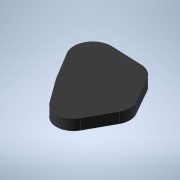
# Autodesk Inventor part: 18650_test
Saved by Autodesk Inventor 2022 (Build 260153000, 153)
## iProperties
Created: 2023-04-04
Part Number: 18650_test
Material: Типовые
Document SubType Name: Modeling
Designer: akapu
Density: 1 g/cm^3
Appearance: По умолчанию
Author: akapu
Autodesk Inventor part; units mm, degrees
ref_plane "YZ Plane" through (0, 0, 0) normal (1, 0, 0) x (0, 1, 0)
ref_plane "XZ Plane" through (0, 0, 0) normal (0, 1, 0) x (-1, 0, 0)
ref_plane "XY Plane" through (0, 0, 0) normal (0, 0, 1) x (1, 0, 0)
sketch "Эскиз1" plane through (0, 0, 0) normal (0, 1, 0) x (-1, 0, 0)
  circle A0 centre (0, 0) radius 9.25
  circle A1 centre (-8.7835, -16.5654) radius 9.5
  circle A2 centre (0.9548, -33.1704) radius 9.75
  circle A3 centre (10.7082, -15.9968) radius 10
  circle A4 centre (20.9526, -33.4643) radius 10.25
  line L0 (19.271, -10.8317) -> (29.7295, -28.1701)
  line L1 (7.4805, 5.4411) -> (18.7952, -10.1146)
  line L2 (-8.1138, 4.4418) -> (-17.1166, -12.0036)
  line L3 (-17.04, -21.2645) -> (-7.5189, -37.9932)
  line L4 (20.5459, -43.7062) -> (0.5679, -42.9128)
  line L5 (9.0979, 6.6175) -> (20.4126, -8.9381)
  line L6 (20.9836, -9.7987) -> (31.4421, -27.1371)
  circle A5 centre (20.9526, -33.4643) radius 12.25
  circle A6 centre (10.7082, -15.9968) radius 12
  circle A7 centre (0, 0) radius 11.25
  line L7 (-9.8681, 5.4022) -> (-18.8709, -11.0432)
  circle A8 centre (-8.7835, -16.5654) radius 11.5
  line L8 (-18.7781, -22.2538) -> (-9.2571, -38.9825)
  circle A9 centre (0.9548, -33.1704) radius 11.75
  line L9 (20.4665, -45.7046) -> (0.4885, -44.9112)
  point P0 (0.7124, -16.2884)
  point P1 (-3.9776, -24.7601)
  point P2 (5.7698, -24.6923)
  point P3 (10.7037, -33.3137)
  point P4 (15.7672, -24.6227)
  point P5 (5.1455, -7.6868)
  point P6 (-4.3332, -8.1723)
  point P7 (0.4885, -44.9112)
  dimension "d0" = 18.5
  dimension "d1" = 19
  dimension "d2" = 19.5
  dimension "d3" = 20
  dimension "d4" = 20.5
  dimension "d5" = 2
  dimension "d6" = 2
  dimension "d7" = 2
  dimension "d8" = 2
  dimension "d9" = 2
  dimension "d10" = 2
  dimension "d11" = 2
  dimension "d12" = 2
  dimension "d13" = 2
  dimension "d14" = 2
  constraints: 20 end point, 17 tangent, 10 centre point, 10 point on circle, 5 parallel, 1 coincident
  measures "d0" diameter of A0
  measures "d1" diameter of A1
  measures "d2" diameter of A2
  measures "d3" diameter of A3
  measures "d4" diameter of A4
  measures "d5" distance between parallel lines of L1 L5
  measures "d6" distance between parallel lines of L0 L6
  measures "d7" radial gap between concentric circles of A4 A5
  measures "d8" radial gap between concentric circles of A3 A6
  measures "d9" radial gap between concentric circles of A0 A7
  measures "d10" distance between parallel lines of L2 L7
  measures "d11" radial gap between concentric circles of A1 A8
  measures "d12" distance between parallel lines of L3 L8
  measures "d13" radial gap between concentric circles of A2 A9
  measures "d14" distance between parallel lines of L4 L9
extrude "Выдавливание1" add sketch "Эскиз1" along normal blind 5 contours A0 L1 A7 A6 | A0 L2 A7 L1 | A6 A7 A3 A0 | A0 A8 A7 L2 | A7 L5 A6 L1 | L1 A6 A7 | A3 A7 A8 A6 A0 | A6 L1 A3 A7 | A6 A8 A0 | A0 A1 A7 A8 | A7 A8 L2 | L2 A8 L7 A7 | A6 L0 A3 L1 | A3 A8 A7 | A8 A6 A7 A1 A0 | A8 A7 A6 | A7 A1 L2 A8 | L2 A1 L3 A8 | A3 A1 A6 A7 A8 | A6 A1 A7 | L0 A6 A5 A3 | L6 A5 L0 A6 | A3 A8 A9 A6 A1 | A1 A9 A8 L3 | A8 L3 A9 L8 | L0 A5 A6 | A5 L4 A4 L0 | A3 A9 A8 | A6 A9 A1 | A1 A2 A8 A9 | A8 A9 L3 | A9 L3 A2 L4 | A5 A6 A4 A3 | L0 A4 A6 A5 | A3 A2 A6 A8 A9 | A8 A6 A9 | A9 A6 A8 A2 A1 | A8 A2 L3 A9 | A9 L4 A5 L9 | A4 A6 A9 A5 A3 | A5 A9 A3 | A3 A9 A5 A6 A2 | A6 A2 A8 | A9 A5 L4 | L4 A2 A5 A9 | A4 A9 A6 | A9 A6 A5 | A5 A9 A4 L4 | A6 A5 A2 | A2 A5 A6 A9 A4 | A5 A2 A4 A9 picked at (0.4928, -9.3459) picked at (11.9874, -28.1937)
sketch "Эскиз2" plane through (0, 5, 0) normal (0, 1, 0) x (1, 0, 0)
  arc A0 (-20.9836, 9.7987) -> (-20.4126, 8.9381) centre (-10.7082, 15.9968) ccw projected
  line L0 (-20.4126, 8.9381) -> (-9.0979, -6.6175) projected
  arc A1 (-9.0979, -6.6175) -> (9.8681, -5.4022) centre (0, 0) ccw projected
  line L1 (9.8681, -5.4022) -> (18.8709, 11.0432) projected
  arc A2 (18.8709, 11.0432) -> (18.7781, 22.2538) centre (8.7835, 16.5654) ccw projected
  line L2 (18.7781, 22.2538) -> (9.2571, 38.9825) projected
  arc A3 (9.2571, 38.9825) -> (-0.4885, 44.9112) centre (-0.9548, 33.1704) ccw projected
  line L3 (-0.4885, 44.9112) -> (-20.4665, 45.7046) projected
  arc A4 (-20.4665, 45.7046) -> (-31.4421, 27.1371) centre (-20.9526, 33.4643) ccw projected
  line L4 (-31.4421, 27.1371) -> (-20.9836, 9.7987) projected
  arc A5 (-10.7037, 33.3137) -> (-15.7672, 24.6227) centre (-20.9526, 33.4643) ccw projected
  arc A6 (3.9776, 24.7601) -> (-10.7037, 33.3137) centre (-0.9548, 33.1704) ccw projected
  arc A7 (4.3332, 8.1723) -> (3.9776, 24.7601) centre (8.7835, 16.5654) ccw projected
  arc A8 (-5.1455, 7.6868) -> (4.3332, 8.1723) centre (0, 0) ccw projected
  arc A9 (-15.7672, 24.6227) -> (-5.1455, 7.6868) centre (-10.7082, 15.9968) ccw projected
  arc A10 (4.3332, 8.1723) -> (-5.1455, 7.6868) centre (0, 0) ccw projected
  arc A11 (-0.7124, 16.2884) -> (4.3332, 8.1723) centre (8.7835, 16.5654) ccw projected
  arc A12 (-5.1455, 7.6868) -> (-0.7124, 16.2884) centre (-10.7082, 15.9968) ccw projected
  arc A13 (3.9776, 24.7601) -> (-0.7124, 16.2884) centre (8.7835, 16.5654) ccw projected
  arc A14 (-5.7698, 24.6923) -> (3.9776, 24.7601) centre (-0.9548, 33.1704) ccw projected
  arc A15 (-0.7124, 16.2884) -> (-5.7698, 24.6923) centre (-10.7082, 15.9968) ccw projected
  arc A16 (-10.7037, 33.3137) -> (-5.7698, 24.6923) centre (-0.9548, 33.1704) ccw projected
  arc A17 (-15.7672, 24.6227) -> (-10.7037, 33.3137) centre (-20.9526, 33.4643) ccw projected
  arc A18 (-5.7698, 24.6923) -> (-15.7672, 24.6227) centre (-10.7082, 15.9968) ccw projected
extrude "Выдавливание2" add sketch "Эскиз2" along normal blind 2 contours L4 A4 L3 A3 L2 A2 L1 A1 L0 A0 | A17 A5 | A6 A14 A16 | A16 A18 A17 | A18 A15 A12 A9 | A7 A11 A13 | A13 A15 A14 | A10 A8 | A12 A11 A10
sketch "Эскиз3" plane through (0, 5, 0) normal (0, -1, 0) x (1, 0, 0)
  arc A0 (-5.1455, -7.6868) -> (4.3332, -8.1723) centre (0, 0) ccw projected
  arc A1 (4.3332, -8.1723) -> (-5.1455, -7.6868) centre (0, 0) ccw projected
  arc A2 (3.9776, -24.7601) -> (4.3332, -8.1723) centre (8.7835, -16.5654) ccw projected
  arc A3 (4.3332, -8.1723) -> (-0.7124, -16.2884) centre (8.7835, -16.5654) ccw projected
  arc A4 (-0.7124, -16.2884) -> (3.9776, -24.7601) centre (8.7835, -16.5654) ccw projected
  arc A5 (-5.7698, -24.6923) -> (-0.7124, -16.2884) centre (-10.7082, -15.9968) ccw projected
  arc A6 (-0.7124, -16.2884) -> (-5.1455, -7.6868) centre (-10.7082, -15.9968) ccw projected
  arc A7 (-5.1455, -7.6868) -> (-15.7672, -24.6227) centre (-10.7082, -15.9968) ccw projected
  arc A8 (-15.7672, -24.6227) -> (-5.7698, -24.6923) centre (-10.7082, -15.9968) ccw projected
  arc A9 (-5.7698, -24.6923) -> (-10.7037, -33.3137) centre (-0.9548, -33.1704) ccw projected
  arc A10 (-10.7037, -33.3137) -> (3.9776, -24.7601) centre (-0.9548, -33.1704) ccw projected
  arc A11 (3.9776, -24.7601) -> (-5.7698, -24.6923) centre (-0.9548, -33.1704) ccw projected
  arc A12 (-15.7672, -24.6227) -> (-10.7037, -33.3137) centre (-20.9526, -33.4643) ccw projected
  arc A13 (-10.7037, -33.3137) -> (-15.7672, -24.6227) centre (-20.9526, -33.4643) ccw projected
  line L0 (-5.2971, 2.241) -> (2.1639, 2.241) construction
  line L1 (2.1639, 2.241) -> (2.1639, -1.4354) construction
  line L2 (2.1639, -1.4354) -> (-5.2971, -1.4354) construction
  line L3 (-5.2971, -1.4354) -> (-5.2971, 2.241) construction
  line L4 (6.0817, -14.3017) -> (10.8583, -14.3017) construction
  line L5 (10.8583, -14.3017) -> (10.8583, -18.5083) construction
  line L6 (10.8583, -18.5083) -> (6.0817, -18.5083) construction
  line L7 (6.0817, -18.5083) -> (6.0817, -14.3017) construction
  line L8 (-6.2539, -35.262) -> (-6.2539, -31.0554) construction
  line L9 (-6.2539, -31.0554) -> (-1.4773, -31.0554) construction
  line L10 (-1.4773, -31.0554) -> (-1.4773, -35.262) construction
  line L11 (-1.4773, -35.262) -> (-6.2539, -35.262) construction
  line L12 (-13.4168, -17.9297) -> (-13.4168, -13.7231) construction
  line L13 (-13.4168, -13.7231) -> (-8.6402, -13.7231) construction
  line L14 (-8.6402, -13.7231) -> (-8.6402, -17.9297) construction
  line L15 (-8.6402, -17.9297) -> (-13.4168, -17.9297) construction
  line L16 (-26.2508, -35.3972) -> (-26.2508, -31.1906) construction
  line L17 (-26.2508, -31.1906) -> (-21.4742, -31.1906) construction
  line L18 (-21.4742, -31.1906) -> (-21.4742, -35.3972) construction
  line L19 (-21.4742, -35.3972) -> (-26.2508, -35.3972) construction
  spline S0 degree 2 poles (-2.4464, -1.59) (-2.4464, -1.6501) (-2.4652, -1.7289) (-2.4952, -1.7778) (-2.5365, -1.8003) (-2.5553, -1.8003) knots 0 0 0 1 2 3 4 4 4
  line L20 (-2.5553, -1.8003) -> (-4.6361, -1.8003)
  spline S1 degree 2 poles (-4.6361, -1.8003) (-4.6586, -1.8003) (-4.6962, -1.7778) (-4.73, -1.7289) (-4.7487, -1.6501) (-4.7487, -1.59) knots 0 0 0 1 2 3 4 4 4
  spline S2 degree 2 poles (-4.7487, -1.59) (-4.7487, -1.5374) (-4.73, -1.4548) (-4.7037, -1.4022) (-4.6624, -1.3759) (-4.6361, -1.3759) knots 0 0 0 1 2 3 4 4 4
  line L21 (-4.6361, -1.3759) -> (-3.806, -1.3759)
  line L22 (-3.806, -1.3759) -> (-3.806, 1.6551)
  line L23 (-3.806, 1.6551) -> (-4.576, 1.1969)
  spline S3 degree 2 poles (-4.576, 1.1969) (-4.6361, 1.1668) (-4.7037, 1.1556) (-4.7487, 1.1931) (-4.7638, 1.287) (-4.7638, 1.3584) knots 0 0 0 1 2 3 4 4 4
  spline S4 degree 2 poles (-4.7638, 1.3584) (-4.7638, 1.4072) (-4.7562, 1.4823) (-4.7375, 1.5311) (-4.7037, 1.5687) (-4.6736, 1.5875) knots 0 0 0 1 2 3 4 4 4
  line L24 (-4.6736, 1.5875) -> (-3.7572, 2.1734)
  spline S5 degree 2 poles (-3.7572, 2.1734) (-3.7459, 2.1847) (-3.7084, 2.1959) (-3.652, 2.2072) (-3.5769, 2.211) (-3.5243, 2.211) knots 0 0 0 1 2 3 4 4 4
  spline S6 degree 2 poles (-3.5243, 2.211) (-3.4492, 2.211) (-3.3516, 2.1997) (-3.2952, 2.1772) (-3.2764, 2.1434) (-3.2764, 2.1246) knots 0 0 0 1 2 3 4 4 4
  line L25 (-3.2764, 2.1246) -> (-3.2764, -1.3759)
  line L26 (-3.2764, -1.3759) -> (-2.5553, -1.3759)
  spline S7 degree 2 poles (-2.5553, -1.3759) (-2.5328, -1.3759) (-2.4877, -1.4022) (-2.4614, -1.4548) (-2.4464, -1.5374) (-2.4464, -1.59) knots 0 0 0 1 2 3 4 4 4
  spline S8 degree 2 poles (0.8287, -0.7787) (0.8287, -1.0379) (0.6447, -1.4397) (0.2954, -1.7177) (-0.2154, -1.8604) (-0.5422, -1.8604) knots 0 0 0 1 2 3 4 4 4
  spline S9 degree 2 poles (-0.5422, -1.8604) (-0.8501, -1.8604) (-1.3347, -1.7327) (-1.6764, -1.4773) (-1.853, -1.1092) (-1.853, -0.8726) knots 0 0 0 1 2 3 4 4 4
  spline S10 degree 2 poles (-1.853, -0.8726) (-1.853, -0.6848) (-1.729, -0.3693) (-1.4999, -0.1064) (-1.1619, 0.1265) (-0.9478, 0.2316) knots 0 0 0 1 2 3 4 4 4
  spline S11 degree 2 poles (-0.9478, 0.2316) (-1.1318, 0.3255) (-1.4173, 0.5396) (-1.6126, 0.7875) (-1.714, 1.0692) (-1.714, 1.2382) knots 0 0 0 1 2 3 4 4 4
  spline S12 degree 2 poles (-1.714, 1.2382) (-1.714, 1.4448) (-1.5638, 1.8128) (-1.2595, 2.0833) (-0.7901, 2.241) (-0.4746, 2.241) knots 0 0 0 1 2 3 4 4 4
  spline S13 degree 2 poles (-0.4746, 2.241) (-0.1741, 2.241) (0.2653, 2.0945) (0.5508, 1.8466) (0.686, 1.5086) (0.686, 1.3133) knots 0 0 0 1 2 3 4 4 4
  spline S14 degree 2 poles (0.686, 1.3133) (0.686, 1.1556) (0.5846, 0.8664) (0.3893, 0.611) (0.1038, 0.3856) (-0.0839, 0.2842) knots 0 0 0 1 2 3 4 4 4
  spline S15 degree 2 poles (-0.0839, 0.2842) (0.1376, 0.179) (0.4794, -0.0501) (0.7085, -0.313) (0.8287, -0.6059) (0.8287, -0.7787) knots 0 0 0 1 2 3 4 4 4
  spline S16 degree 2 poles (0.2916, -0.835) (0.2916, -0.6923) (0.1865, -0.4632) (-0.0239, -0.2604) (-0.3393, -0.0726) (-0.5497, 0.0288) knots 0 0 0 1 2 3 4 4 4
  spline S17 degree 2 poles (-0.5497, 0.0288) (-0.7412, -0.0689) (-1.0342, -0.2604) (-1.222, -0.4632) (-1.3159, -0.6886) (-1.3159, -0.8238) knots 0 0 0 1 2 3 4 4 4
  spline S18 degree 2 poles (-1.3159, -0.8238) (-1.3159, -1.1205) (-0.9065, -1.4473) (-0.5046, -1.4473) knots 0 0 0 1 2 2 2
  spline S19 degree 2 poles (-0.5046, -1.4473) (-0.1102, -1.4473) (0.2916, -1.1167) (0.2916, -0.835) knots 0 0 0 1 2 2 2
  spline S20 degree 2 poles (0.1639, 1.2645) (0.1639, 1.3922) (0.0738, 1.6025) (-0.099, 1.7527) (-0.3506, 1.8279) (-0.5159, 1.8279) knots 0 0 0 1 2 3 4 4 4
  spline S21 degree 2 poles (-0.5159, 1.8279) (-0.8464, 1.8279) (-1.1882, 1.5274) (-1.1882, 1.2645) knots 0 0 0 1 2 2 2
  spline S22 degree 2 poles (-1.1882, 1.2645) (-1.1882, 1.1443) (-1.1055, 0.9377) (-0.929, 0.7537) (-0.6624, 0.5772) (-0.4783, 0.4833) knots 0 0 0 1 2 3 4 4 4
  spline S23 degree 2 poles (-0.4783, 0.4833) (-0.1666, 0.6448) (0.1639, 1.0316) (0.1639, 1.2645) knots 0 0 0 1 2 2 2
  spline S24 degree 2 poles (2.2146, -1.4623) (2.2146, -1.6801) (2.0719, -1.8266) (1.8804, -1.8266) knots 0 0 0 1 2 2 2
  spline S25 degree 2 poles (1.8804, -1.8266) (1.6963, -1.8266) (1.5536, -1.6839) (1.5536, -1.4735) knots 0 0 0 1 2 2 2
  spline S26 degree 2 poles (1.5536, -1.4735) (1.5536, -1.2557) (1.7001, -1.1092) (1.8879, -1.1092) knots 0 0 0 1 2 2 2
  spline S27 degree 2 poles (1.8879, -1.1092) (2.0719, -1.1092) (2.2146, -1.2519) (2.2146, -1.4623) knots 0 0 0 1 2 2 2
  spline S28 degree 2 poles (5.5048, -0.5233) (5.5048, -0.8426) (5.2907, -1.3421) (4.8963, -1.6801) (4.3517, -1.8604) (4.0212, -1.8604) knots 0 0 0 1 2 3 4 4 4
  spline S29 degree 2 poles (4.0212, -1.8604) (3.8334, -1.8604) (3.5029, -1.8078) (3.2438, -1.7327) (3.0785, -1.6576) (3.0334, -1.6125) (3.0146, -1.5787) (2.9996, -1.5261) (2.9921, -1.4435) (2.9921, -1.3909) knots 0 0 0 1 2 3 4 5 6 7 8 8 8
  spline S30 degree 2 poles (2.9921, -1.3909) (2.9921, -1.3383) (2.9996, -1.2519) (3.0259, -1.2031) (3.0597, -1.1768) (3.0822, -1.1768) knots 0 0 0 1 2 3 4 4 4
  spline S31 degree 2 poles (3.0822, -1.1768) (3.1123, -1.1768) (3.24, -1.2557) (3.4578, -1.3458) (3.7808, -1.4247) (4.0024, -1.4247) knots 0 0 0 1 2 3 4 4 4
  spline S32 degree 2 poles (4.0024, -1.4247) (4.209, -1.4247) (4.5545, -1.3271) (4.8024, -1.1167) (4.9452, -0.8012) (4.9452, -0.5721) knots 0 0 0 1 2 3 4 4 4
  spline S33 degree 2 poles (4.9452, -0.5721) (4.9452, -0.3806) (4.825, -0.0876) (4.5771, 0.1077) (4.194, 0.2016) (3.9311, 0.2016) knots 0 0 0 1 2 3 4 4 4
  spline S34 degree 2 poles (3.9311, 0.2016) (3.7433, 0.2016) (3.4729, 0.164) (3.3564, 0.164) knots 0 0 0 1 2 2 2
  spline S35 degree 2 poles (3.3564, 0.164) (3.27, 0.164) (3.1949, 0.2429) (3.1949, 0.3593) knots 0 0 0 1 2 2 2
  line L27 (3.1949, 0.3593) -> (3.1949, 1.9819)
  spline S36 degree 2 poles (3.1949, 1.9819) (3.1949, 2.0833) (3.2888, 2.1809) (3.379, 2.1809) knots 0 0 0 1 2 2 2
  line L28 (3.379, 2.1809) -> (5.1405, 2.1809)
  spline S37 degree 2 poles (5.1405, 2.1809) (5.163, 2.1809) (5.2118, 2.1546) (5.2419, 2.0983) (5.2569, 2.0119) (5.2569, 1.9518) knots 0 0 0 1 2 3 4 4 4
  spline S38 degree 2 poles (5.2569, 1.9518) (5.2569, 1.8429) (5.1968, 1.7189) (5.1442, 1.7189) knots 0 0 0 1 2 2 2
  line L29 (5.1442, 1.7189) -> (3.7245, 1.7189)
  line L30 (3.7245, 1.7189) -> (3.7245, 0.5997)
  spline S39 degree 2 poles (3.7245, 0.5997) (3.8297, 0.6147) (4.0438, 0.6222) (4.1865, 0.6222) knots 0 0 0 1 2 2 2
  spline S40 degree 2 poles (4.1865, 0.6222) (4.517, 0.6222) (5.009, 0.4607) (5.3358, 0.1603) (5.5048, -0.2642) (5.5048, -0.5233) knots 0 0 0 1 2 3 4 4 4
  spline S41 degree 2 poles (8.9324, -18.1327) (8.9324, -18.1928) (8.9136, -18.2716) (8.8836, -18.3205) (8.8423, -18.343) (8.8235, -18.343) knots 0 0 0 1 2 3 4 4 4
  line L31 (8.8235, -18.343) -> (6.7427, -18.343)
  spline S42 degree 2 poles (6.7427, -18.343) (6.7202, -18.343) (6.6826, -18.3205) (6.6488, -18.2716) (6.6301, -18.1928) (6.6301, -18.1327) knots 0 0 0 1 2 3 4 4 4
  spline S43 degree 2 poles (6.6301, -18.1327) (6.6301, -18.0801) (6.6488, -17.9975) (6.6751, -17.9449) (6.7165, -17.9186) (6.7427, -17.9186) knots 0 0 0 1 2 3 4 4 4
  line L32 (6.7427, -17.9186) -> (7.5728, -17.9186)
  line L33 (7.5728, -17.9186) -> (7.5728, -14.8876)
  line L34 (7.5728, -14.8876) -> (6.8028, -15.3458)
  spline S44 degree 2 poles (6.8028, -15.3458) (6.7427, -15.3759) (6.6751, -15.3871) (6.6301, -15.3496) (6.615, -15.2557) (6.615, -15.1843) knots 0 0 0 1 2 3 4 4 4
  spline S45 degree 2 poles (6.615, -15.1843) (6.615, -15.1355) (6.6226, -15.0604) (6.6413, -15.0115) (6.6751, -14.974) (6.7052, -14.9552) knots 0 0 0 1 2 3 4 4 4
  line L35 (6.7052, -14.9552) -> (7.6216, -14.3693)
  spline S46 degree 2 poles (7.6216, -14.3693) (7.6329, -14.358) (7.6704, -14.3468) (7.7268, -14.3355) (7.8019, -14.3317) (7.8545, -14.3317) knots 0 0 0 1 2 3 4 4 4
  spline S47 degree 2 poles (7.8545, -14.3317) (7.9296, -14.3317) (8.0272, -14.343) (8.0836, -14.3655) (8.1024, -14.3993) (8.1024, -14.4181) knots 0 0 0 1 2 3 4 4 4
  line L36 (8.1024, -14.4181) -> (8.1024, -17.9186)
  line L37 (8.1024, -17.9186) -> (8.8235, -17.9186)
  spline S48 degree 2 poles (8.8235, -17.9186) (8.846, -17.9186) (8.8911, -17.9449) (8.9174, -17.9975) (8.9324, -18.0801) (8.9324, -18.1327) knots 0 0 0 1 2 3 4 4 4
  spline S49 degree 2 poles (12.1474, -16.1946) (12.1474, -16.4538) (12.0873, -16.9834) (11.9371, -17.4716) (11.6892, -17.8998) (11.3099, -18.2228) (10.7916, -18.4031) (10.446, -18.4031) knots 0 0 0 1 2 3 4 5 6 6 6
  spline S50 degree 2 poles (10.446, -18.4031) (10.3146, -18.4031) (10.0629, -18.3693) (9.8639, -18.3205) (9.7287, -18.2641) (9.6648, -18.2078) (9.6385, -18.1139) (9.6385, -18.035) knots 0 0 0 1 2 3 4 5 6 6 6
  spline S51 degree 2 poles (9.6385, -18.035) (9.6385, -17.9674) (9.646, -17.8848) (9.6648, -17.8435) (9.6986, -17.8284) (9.7249, -17.8284) knots 0 0 0 1 2 3 4 4 4
  spline S52 degree 2 poles (9.7249, -17.8284) (9.7587, -17.8284) (9.8826, -17.8735) (10.0704, -17.9299) (10.3221, -17.9749) (10.4798, -17.9749) knots 0 0 0 1 2 3 4 4 4
  spline S53 degree 2 poles (10.4798, -17.9749) (10.7803, -17.9749) (11.2085, -17.7458) (11.4789, -17.3552) (11.6141, -16.8482) (11.6179, -16.5627) knots 0 0 0 1 2 3 4 4 4
  spline S54 degree 2 poles (11.6179, -16.5627) (11.4564, -16.6604) (11.0019, -16.8069) (10.7052, -16.8069) knots 0 0 0 1 2 2 2
  spline S55 degree 2 poles (10.7052, -16.8069) (10.3709, -16.8069) (9.9202, -16.6266) (9.646, -16.3111) (9.5258, -15.8792) (9.5258, -15.6238) knots 0 0 0 1 2 3 4 4 4
  spline S56 degree 2 poles (9.5258, -15.6238) (9.5258, -15.3571) (9.6798, -14.8801) (10.0066, -14.5158) (10.5099, -14.3017) (10.8629, -14.3017) knots 0 0 0 1 2 3 4 4 4
  spline S57 degree 2 poles (10.8629, -14.3017) (11.1108, -14.3017) (11.4939, -14.4294) (11.7794, -14.666) (11.9747, -15.0003) (12.0949, -15.4247) (12.1474, -15.9205) (12.1474, -16.1946) knots 0 0 0 1 2 3 4 5 6 6 6
  spline S58 degree 2 poles (11.6103, -16.1383) (11.6103, -15.7439) (11.5052, -15.2031) (11.3024, -14.8688) (11.0057, -14.7223) (10.8141, -14.7223) knots 0 0 0 1 2 3 4 4 4
  spline S59 degree 2 poles (10.8141, -14.7223) (10.615, -14.7223) (10.3296, -14.8688) (10.1493, -15.1092) (10.0629, -15.4172) (10.0629, -15.5824) knots 0 0 0 1 2 3 4 4 4
  spline S60 degree 2 poles (10.0629, -15.5824) (10.0629, -15.7627) (10.138, -16.0669) (10.3108, -16.2773) (10.5888, -16.39) (10.7916, -16.39) knots 0 0 0 1 2 3 4 4 4
  spline S61 degree 2 poles (10.7916, -16.39) (11.0244, -16.39) (11.4526, -16.251) (11.6103, -16.1383) knots 0 0 0 1 2 2 2
  spline S62 degree 2 poles (-10.5736, -17.5353) (-10.5736, -17.5916) (-10.5887, -17.678) (-10.615, -17.7381) (-10.6638, -17.7644) (-10.6901, -17.7644) knots 0 0 0 1 2 3 4 4 4
  line L38 (-10.6901, -17.7644) -> (-12.891, -17.7644)
  spline S63 degree 2 poles (-12.891, -17.7644) (-12.9361, -17.7644) (-12.9999, -17.7419) (-13.045, -17.693) (-13.0675, -17.5991) (-13.0675, -17.5315) knots 0 0 0 1 2 3 4 4 4
  spline S64 degree 2 poles (-13.0675, -17.5315) (-13.0675, -17.4714) (-13.0563, -17.3775) (-13.0262, -17.3062) (-12.9774, -17.2386) (-12.9398, -17.1973) knots 0 0 0 1 2 3 4 4 4
  line L39 (-12.9398, -17.1973) -> (-12.1436, -16.3785)
  spline S65 degree 2 poles (-12.1436, -16.3785) (-11.8657, -16.0968) (-11.5314, -15.6461) (-11.3511, -15.278) (-11.2948, -14.9775) (-11.2948, -14.8423) knots 0 0 0 1 2 3 4 4 4
  spline S66 degree 2 poles (-11.2948, -14.8423) (-11.2948, -14.7109) (-11.3849, -14.4743) (-11.5539, -14.2977) (-11.8056, -14.1926) (-11.9708, -14.1926) knots 0 0 0 1 2 3 4 4 4
  spline S67 degree 2 poles (-11.9708, -14.1926) (-12.1661, -14.1926) (-12.4741, -14.2977) (-12.707, -14.4179) (-12.861, -14.5231) (-12.8985, -14.5231) knots 0 0 0 1 2 3 4 4 4
  spline S68 degree 2 poles (-12.8985, -14.5231) (-12.9211, -14.5231) (-12.9586, -14.4968) (-12.9812, -14.4442) (-12.9924, -14.3503) (-12.9924, -14.2865) knots 0 0 0 1 2 3 4 4 4
  spline S69 degree 2 poles (-12.9924, -14.2865) (-12.9924, -14.2414) (-12.9849, -14.1738) (-12.9699, -14.1212) (-12.9473, -14.0799) (-12.8722, -14.016) (-12.6919, -13.9034) (-12.4178, -13.7982) (-12.0873, -13.7231) (-11.907, -13.7231) knots 0 0 0 1 2 3 4 5 6 7 8 8 8
  spline S70 degree 2 poles (-11.907, -13.7231) (-11.6178, -13.7231) (-11.1821, -13.8846) (-10.8966, -14.17) (-10.7539, -14.5456) (-10.7539, -14.7559) knots 0 0 0 1 2 3 4 4 4
  spline S71 degree 2 poles (-10.7539, -14.7559) (-10.7539, -14.9475) (-10.8215, -15.3268) (-11.0394, -15.7663) (-11.4525, -16.3034) (-11.7981, -16.6564) knots 0 0 0 1 2 3 4 4 4
  line L40 (-11.7981, -16.6564) -> (-12.429, -17.3137)
  line L41 (-12.429, -17.3137) -> (-10.6938, -17.3137)
  spline S72 degree 2 poles (-10.6938, -17.3137) (-10.6675, -17.3137) (-10.6225, -17.34) (-10.5887, -17.3963) (-10.5736, -17.479) (-10.5736, -17.5353) knots 0 0 0 1 2 3 4 4 4
  spline S73 degree 2 poles (-7.2497, -15.7663) (-7.2497, -16.2245) (-7.3924, -16.9794) (-7.7304, -17.524) (-8.2713, -17.8245) (-8.6694, -17.8245) knots 0 0 0 1 2 3 4 4 4
  spline S74 degree 2 poles (-8.6694, -17.8245) (-9.0412, -17.8245) (-9.5558, -17.5578) (-9.8713, -17.0358) (-10.0027, -16.2771) (-10.0027, -15.7813) knots 0 0 0 1 2 3 4 4 4
  spline S75 degree 2 poles (-10.0027, -15.7813) (-10.0027, -15.3268) (-9.8563, -14.5682) (-9.522, -14.0236) (-8.9812, -13.7231) (-8.5868, -13.7231) knots 0 0 0 1 2 3 4 4 4
  spline S76 degree 2 poles (-8.5868, -13.7231) (-8.2112, -13.7231) (-7.6966, -13.9898) (-7.3812, -14.5118) (-7.2497, -15.2705) (-7.2497, -15.7663) knots 0 0 0 1 2 3 4 4 4
  spline S77 degree 2 poles (-7.7905, -15.8001) (-7.7905, -15.5034) (-7.8319, -15.0301) (-7.9182, -14.6658) (-8.0497, -14.4067) (-8.2337, -14.2339) (-8.4704, -14.1588) (-8.6168, -14.1588) knots 0 0 0 1 2 3 4 5 6 6 6
  spline S78 degree 2 poles (-8.6168, -14.1588) (-8.8797, -14.1588) (-9.2065, -14.4067) (-9.3943, -14.8348) (-9.4619, -15.4132) (-9.4619, -15.7475) knots 0 0 0 1 2 3 4 4 4
  spline S79 degree 2 poles (-9.4619, -15.7475) (-9.4619, -16.1907) (-9.368, -16.8179) (-9.1689, -17.2085) (-8.8572, -17.3888) (-8.6356, -17.3888) knots 0 0 0 1 2 3 4 4 4
  spline S80 degree 2 poles (-8.6356, -17.3888) (-8.4628, -17.3888) (-8.2037, -17.2799) (-8.0159, -17.0733) (-7.8919, -16.7841) (-7.8168, -16.4311) (-7.7905, -16.0217) (-7.7905, -15.8001) knots 0 0 0 1 2 3 4 5 6 6 6
  spline S81 degree 2 poles (-3.4032, -34.8864) (-3.4032, -34.9465) (-3.422, -35.0254) (-3.452, -35.0742) (-3.4934, -35.0967) (-3.5121, -35.0967) knots 0 0 0 1 2 3 4 4 4
  line L42 (-3.5121, -35.0967) -> (-5.5929, -35.0967)
  spline S82 degree 2 poles (-5.5929, -35.0967) (-5.6154, -35.0967) (-5.653, -35.0742) (-5.6868, -35.0254) (-5.7056, -34.9465) (-5.7056, -34.8864) knots 0 0 0 1 2 3 4 4 4
  spline S83 degree 2 poles (-5.7056, -34.8864) (-5.7056, -34.8338) (-5.6868, -34.7512) (-5.6605, -34.6986) (-5.6192, -34.6723) (-5.5929, -34.6723) knots 0 0 0 1 2 3 4 4 4
  line L43 (-5.5929, -34.6723) -> (-4.7628, -34.6723)
  line L44 (-4.7628, -34.6723) -> (-4.7628, -31.6413)
  line L45 (-4.7628, -31.6413) -> (-5.5328, -32.0996)
  spline S84 degree 2 poles (-5.5328, -32.0996) (-5.5929, -32.1296) (-5.6605, -32.1409) (-5.7056, -32.1033) (-5.7206, -32.0094) (-5.7206, -31.9381) knots 0 0 0 1 2 3 4 4 4
  spline S85 degree 2 poles (-5.7206, -31.9381) (-5.7206, -31.8892) (-5.7131, -31.8141) (-5.6943, -31.7653) (-5.6605, -31.7277) (-5.6304, -31.7089) knots 0 0 0 1 2 3 4 4 4
  line L46 (-5.6304, -31.7089) -> (-4.714, -31.123)
  spline S86 degree 2 poles (-4.714, -31.123) (-4.7027, -31.1118) (-4.6652, -31.1005) (-4.6088, -31.0892) (-4.5337, -31.0855) (-4.4811, -31.0855) knots 0 0 0 1 2 3 4 4 4
  spline S87 degree 2 poles (-4.4811, -31.0855) (-4.406, -31.0855) (-4.3084, -31.0967) (-4.252, -31.1193) (-4.2333, -31.1531) (-4.2333, -31.1719) knots 0 0 0 1 2 3 4 4 4
  line L47 (-4.2333, -31.1719) -> (-4.2333, -34.6723)
  line L48 (-4.2333, -34.6723) -> (-3.5121, -34.6723)
  spline S88 degree 2 poles (-3.5121, -34.6723) (-3.4896, -34.6723) (-3.4445, -34.6986) (-3.4182, -34.7512) (-3.4032, -34.8338) (-3.4032, -34.8864) knots 0 0 0 1 2 3 4 4 4
  spline S89 degree 2 poles (-0.1882, -32.9484) (-0.1882, -33.2075) (-0.2483, -33.7371) (-0.3985, -34.2254) (-0.6464, -34.6536) (-1.0257, -34.9766) (-1.5441, -35.1568) (-1.8896, -35.1568) knots 0 0 0 1 2 3 4 5 6 6 6
  spline S90 degree 2 poles (-1.8896, -35.1568) (-2.0211, -35.1568) (-2.2727, -35.123) (-2.4718, -35.0742) (-2.607, -35.0179) (-2.6708, -34.9615) (-2.6971, -34.8676) (-2.6971, -34.7888) knots 0 0 0 1 2 3 4 5 6 6 6
  spline S91 degree 2 poles (-2.6971, -34.7888) (-2.6971, -34.7212) (-2.6896, -34.6385) (-2.6708, -34.5972) (-2.637, -34.5822) (-2.6107, -34.5822) knots 0 0 0 1 2 3 4 4 4
  spline S92 degree 2 poles (-2.6107, -34.5822) (-2.5769, -34.5822) (-2.453, -34.6273) (-2.2652, -34.6836) (-2.0135, -34.7287) (-1.8558, -34.7287) knots 0 0 0 1 2 3 4 4 4
  spline S93 degree 2 poles (-1.8558, -34.7287) (-1.5553, -34.7287) (-1.1272, -34.4996) (-0.8567, -34.1089) (-0.7215, -33.6019) (-0.7178, -33.3165) knots 0 0 0 1 2 3 4 4 4
  spline S94 degree 2 poles (-0.7178, -33.3165) (-0.8793, -33.4141) (-1.3337, -33.5606) (-1.6304, -33.5606) knots 0 0 0 1 2 2 2
  spline S95 degree 2 poles (-1.6304, -33.5606) (-1.9647, -33.5606) (-2.4154, -33.3803) (-2.6896, -33.0648) (-2.8098, -32.6329) (-2.8098, -32.3775) knots 0 0 0 1 2 3 4 4 4
  spline S96 degree 2 poles (-2.8098, -32.3775) (-2.8098, -32.1108) (-2.6558, -31.6338) (-2.329, -31.2695) (-1.8257, -31.0554) (-1.4727, -31.0554) knots 0 0 0 1 2 3 4 4 4
  spline S97 degree 2 poles (-1.4727, -31.0554) (-1.2248, -31.0554) (-0.8417, -31.1831) (-0.5563, -31.4197) (-0.361, -31.754) (-0.2408, -32.1784) (-0.1882, -32.6742) (-0.1882, -32.9484) knots 0 0 0 1 2 3 4 5 6 6 6
  spline S98 degree 2 poles (-0.7253, -32.892) (-0.7253, -32.4977) (-0.8304, -31.9568) (-1.0333, -31.6226) (-1.33, -31.4761) (-1.5215, -31.4761) knots 0 0 0 1 2 3 4 4 4
  spline S99 degree 2 poles (-1.5215, -31.4761) (-1.7206, -31.4761) (-2.006, -31.6226) (-2.1863, -31.8629) (-2.2727, -32.1709) (-2.2727, -32.3362) knots 0 0 0 1 2 3 4 4 4
  spline S100 degree 2 poles (-2.2727, -32.3362) (-2.2727, -32.5165) (-2.1976, -32.8207) (-2.0248, -33.031) (-1.7469, -33.1437) (-1.5441, -33.1437) knots 0 0 0 1 2 3 4 4 4
  spline S101 degree 2 poles (-1.5441, -33.1437) (-1.3112, -33.1437) (-0.883, -33.0047) (-0.7253, -32.892) knots 0 0 0 1 2 2 2
  spline S102 degree 2 poles (1.2578, -34.7587) (1.2578, -34.9766) (1.1151, -35.123) (0.9235, -35.123) knots 0 0 0 1 2 2 2
  spline S103 degree 2 poles (0.9235, -35.123) (0.7395, -35.123) (0.5968, -34.9803) (0.5968, -34.77) knots 0 0 0 1 2 2 2
  spline S104 degree 2 poles (0.5968, -34.77) (0.5968, -34.5521) (0.7433, -34.4057) (0.9311, -34.4057) knots 0 0 0 1 2 2 2
  spline S105 degree 2 poles (0.9311, -34.4057) (1.1151, -34.4057) (1.2578, -34.5484) (1.2578, -34.7587) knots 0 0 0 1 2 2 2
  spline S106 degree 2 poles (4.548, -33.8197) (4.548, -34.139) (4.3339, -34.6385) (3.9395, -34.9766) (3.3949, -35.1568) (3.0644, -35.1568) knots 0 0 0 1 2 3 4 4 4
  spline S107 degree 2 poles (3.0644, -35.1568) (2.8766, -35.1568) (2.5461, -35.1043) (2.2869, -35.0291) (2.1217, -34.954) (2.0766, -34.9089) (2.0578, -34.8751) (2.0428, -34.8226) (2.0353, -34.7399) (2.0353, -34.6874) knots 0 0 0 1 2 3 4 5 6 7 8 8 8
  spline S108 degree 2 poles (2.0353, -34.6874) (2.0353, -34.6348) (2.0428, -34.5484) (2.0691, -34.4996) (2.1029, -34.4733) (2.1254, -34.4733) knots 0 0 0 1 2 3 4 4 4
  spline S109 degree 2 poles (2.1254, -34.4733) (2.1555, -34.4733) (2.2832, -34.5521) (2.501, -34.6423) (2.824, -34.7212) (3.0456, -34.7212) knots 0 0 0 1 2 3 4 4 4
  spline S110 degree 2 poles (3.0456, -34.7212) (3.2522, -34.7212) (3.5977, -34.6235) (3.8456, -34.4132) (3.9883, -34.0977) (3.9883, -33.8686) knots 0 0 0 1 2 3 4 4 4
  spline S111 degree 2 poles (3.9883, -33.8686) (3.9883, -33.677) (3.8681, -33.3841) (3.6203, -33.1888) (3.2372, -33.0949) (2.9743, -33.0949) knots 0 0 0 1 2 3 4 4 4
  spline S112 degree 2 poles (2.9743, -33.0949) (2.7865, -33.0949) (2.516, -33.1324) (2.3996, -33.1324) knots 0 0 0 1 2 2 2
  spline S113 degree 2 poles (2.3996, -33.1324) (2.3132, -33.1324) (2.2381, -33.0536) (2.2381, -32.9371) knots 0 0 0 1 2 2 2
  line L49 (2.2381, -32.9371) -> (2.2381, -31.3146)
  spline S114 degree 2 poles (2.2381, -31.3146) (2.2381, -31.2132) (2.332, -31.1155) (2.4221, -31.1155) knots 0 0 0 1 2 2 2
  line L50 (2.4221, -31.1155) -> (4.1836, -31.1155)
  spline S115 degree 2 poles (4.1836, -31.1155) (4.2062, -31.1155) (4.255, -31.1418) (4.285, -31.1982) (4.3001, -31.2845) (4.3001, -31.3446) knots 0 0 0 1 2 3 4 4 4
  spline S116 degree 2 poles (4.3001, -31.3446) (4.3001, -31.4536) (4.24, -31.5775) (4.1874, -31.5775) knots 0 0 0 1 2 2 2
  line L51 (4.1874, -31.5775) -> (2.7677, -31.5775)
  line L52 (2.7677, -31.5775) -> (2.7677, -32.6967)
  spline S117 degree 2 poles (2.7677, -32.6967) (2.8728, -32.6817) (3.0869, -32.6742) (3.2297, -32.6742) knots 0 0 0 1 2 2 2
  spline S118 degree 2 poles (3.2297, -32.6742) (3.5602, -32.6742) (4.0522, -32.8357) (4.3789, -33.1362) (4.548, -33.5606) (4.548, -33.8197) knots 0 0 0 1 2 3 4 4 4
  spline S119 degree 2 poles (-23.4076, -35.0028) (-23.4076, -35.0591) (-23.4227, -35.1455) (-23.449, -35.2056) (-23.4978, -35.2319) (-23.5241, -35.2319) knots 0 0 0 1 2 3 4 4 4
  line L53 (-23.5241, -35.2319) -> (-25.725, -35.2319)
  spline S120 degree 2 poles (-25.725, -35.2319) (-25.7701, -35.2319) (-25.8339, -35.2094) (-25.879, -35.1606) (-25.9015, -35.0667) (-25.9015, -34.9991) knots 0 0 0 1 2 3 4 4 4
  spline S121 degree 2 poles (-25.9015, -34.9991) (-25.9015, -34.939) (-25.8903, -34.8451) (-25.8602, -34.7737) (-25.8114, -34.7061) (-25.7738, -34.6648) knots 0 0 0 1 2 3 4 4 4
  line L54 (-25.7738, -34.6648) -> (-24.9776, -33.846)
  spline S122 degree 2 poles (-24.9776, -33.846) (-24.6997, -33.5643) (-24.3654, -33.1136) (-24.1851, -32.7455) (-24.1288, -32.4451) (-24.1288, -32.3099) knots 0 0 0 1 2 3 4 4 4
  spline S123 degree 2 poles (-24.1288, -32.3099) (-24.1288, -32.1784) (-24.2189, -31.9418) (-24.3879, -31.7653) (-24.6396, -31.6601) (-24.8048, -31.6601) knots 0 0 0 1 2 3 4 4 4
  spline S124 degree 2 poles (-24.8048, -31.6601) (-25.0001, -31.6601) (-25.3081, -31.7653) (-25.541, -31.8854) (-25.695, -31.9906) (-25.7325, -31.9906) knots 0 0 0 1 2 3 4 4 4
  spline S125 degree 2 poles (-25.7325, -31.9906) (-25.7551, -31.9906) (-25.7926, -31.9643) (-25.8152, -31.9117) (-25.8264, -31.8178) (-25.8264, -31.754) knots 0 0 0 1 2 3 4 4 4
  spline S126 degree 2 poles (-25.8264, -31.754) (-25.8264, -31.7089) (-25.8189, -31.6413) (-25.8039, -31.5887) (-25.7814, -31.5474) (-25.7062, -31.4836) (-25.526, -31.3709) (-25.2518, -31.2657) (-24.9213, -31.1906) (-24.741, -31.1906) knots 0 0 0 1 2 3 4 5 6 7 8 8 8
  spline S127 degree 2 poles (-24.741, -31.1906) (-24.4518, -31.1906) (-24.0161, -31.3521) (-23.7307, -31.6376) (-23.5879, -32.0131) (-23.5879, -32.2235) knots 0 0 0 1 2 3 4 4 4
  spline S128 degree 2 poles (-23.5879, -32.2235) (-23.5879, -32.415) (-23.6555, -32.7944) (-23.8734, -33.2338) (-24.2865, -33.7709) (-24.6321, -34.1239) knots 0 0 0 1 2 3 4 4 4
  line L55 (-24.6321, -34.1239) -> (-25.263, -34.7812)
  line L56 (-25.263, -34.7812) -> (-23.5278, -34.7812)
  spline S129 degree 2 poles (-23.5278, -34.7812) (-23.5015, -34.7812) (-23.4565, -34.8075) (-23.4227, -34.8638) (-23.4076, -34.9465) (-23.4076, -35.0028) knots 0 0 0 1 2 3 4 4 4
  spline S130 degree 2 poles (-20.0837, -33.2338) (-20.0837, -33.692) (-20.2264, -34.4469) (-20.5645, -34.9915) (-21.1053, -35.292) (-21.5034, -35.292) knots 0 0 0 1 2 3 4 4 4
  spline S131 degree 2 poles (-21.5034, -35.292) (-21.8753, -35.292) (-22.3898, -35.0253) (-22.7053, -34.5033) (-22.8368, -33.7446) (-22.8368, -33.2488) knots 0 0 0 1 2 3 4 4 4
  spline S132 degree 2 poles (-22.8368, -33.2488) (-22.8368, -32.7944) (-22.6903, -32.0357) (-22.356, -31.4911) (-21.8152, -31.1906) (-21.4208, -31.1906) knots 0 0 0 1 2 3 4 4 4
  spline S133 degree 2 poles (-21.4208, -31.1906) (-21.0452, -31.1906) (-20.5307, -31.4573) (-20.2152, -31.9793) (-20.0837, -32.738) (-20.0837, -33.2338) knots 0 0 0 1 2 3 4 4 4
  spline S134 degree 2 poles (-20.6246, -33.2676) (-20.6246, -32.9709) (-20.6659, -32.4976) (-20.7522, -32.1333) (-20.8837, -31.8742) (-21.0677, -31.7014) (-21.3044, -31.6263) (-21.4508, -31.6263) knots 0 0 0 1 2 3 4 5 6 6 6
  spline S135 degree 2 poles (-21.4508, -31.6263) (-21.7138, -31.6263) (-22.0405, -31.8742) (-22.2283, -32.3023) (-22.2959, -32.8807) (-22.2959, -33.215) knots 0 0 0 1 2 3 4 4 4
  spline S136 degree 2 poles (-22.2959, -33.215) (-22.2959, -33.6582) (-22.202, -34.2854) (-22.003, -34.6761) (-21.6912, -34.8563) (-21.4696, -34.8563) knots 0 0 0 1 2 3 4 4 4
  spline S137 degree 2 poles (-21.4696, -34.8563) (-21.2969, -34.8563) (-21.0377, -34.7474) (-20.8499, -34.5408) (-20.726, -34.2516) (-20.6508, -33.8986) (-20.6246, -33.4892) (-20.6246, -33.2676) knots 0 0 0 1 2 3 4 5 6 6 6
  spline S138 degree 2 poles (-18.7391, -34.8939) (-18.7391, -35.1117) (-18.8818, -35.2582) (-19.0734, -35.2582) knots 0 0 0 1 2 2 2
  spline S139 degree 2 poles (-19.0734, -35.2582) (-19.2574, -35.2582) (-19.4001, -35.1155) (-19.4001, -34.9052) knots 0 0 0 1 2 2 2
  spline S140 degree 2 poles (-19.4001, -34.9052) (-19.4001, -34.6873) (-19.2537, -34.5408) (-19.0659, -34.5408) knots 0 0 0 1 2 2 2
  spline S141 degree 2 poles (-19.0659, -34.5408) (-18.8818, -34.5408) (-18.7391, -34.6836) (-18.7391, -34.8939) knots 0 0 0 1 2 2 2
  spline S142 degree 2 poles (-15.449, -33.9549) (-15.449, -34.2742) (-15.663, -34.7737) (-16.0574, -35.1117) (-16.602, -35.292) (-16.9325, -35.292) knots 0 0 0 1 2 3 4 4 4
  spline S143 degree 2 poles (-16.9325, -35.292) (-17.1203, -35.292) (-17.4508, -35.2394) (-17.71, -35.1643) (-17.8753, -35.0892) (-17.9203, -35.0441) (-17.9391, -35.0103) (-17.9541, -34.9577) (-17.9616, -34.8751) (-17.9616, -34.8225) knots 0 0 0 1 2 3 4 5 6 7 8 8 8
  spline S144 degree 2 poles (-17.9616, -34.8225) (-17.9616, -34.7699) (-17.9541, -34.6836) (-17.9278, -34.6347) (-17.894, -34.6084) (-17.8715, -34.6084) knots 0 0 0 1 2 3 4 4 4
  spline S145 degree 2 poles (-17.8715, -34.6084) (-17.8415, -34.6084) (-17.7138, -34.6873) (-17.4959, -34.7775) (-17.1729, -34.8563) (-16.9513, -34.8563) knots 0 0 0 1 2 3 4 4 4
  spline S146 degree 2 poles (-16.9513, -34.8563) (-16.7447, -34.8563) (-16.3992, -34.7587) (-16.1513, -34.5484) (-16.0086, -34.2329) (-16.0086, -34.0038) knots 0 0 0 1 2 3 4 4 4
  spline S147 degree 2 poles (-16.0086, -34.0038) (-16.0086, -33.8122) (-16.1288, -33.5192) (-16.3767, -33.3239) (-16.7598, -33.23) (-17.0227, -33.23) knots 0 0 0 1 2 3 4 4 4
  spline S148 degree 2 poles (-17.0227, -33.23) (-17.2105, -33.23) (-17.4809, -33.2676) (-17.5973, -33.2676) knots 0 0 0 1 2 2 2
  spline S149 degree 2 poles (-17.5973, -33.2676) (-17.6837, -33.2676) (-17.7588, -33.1887) (-17.7588, -33.0723) knots 0 0 0 1 2 2 2
  line L57 (-17.7588, -33.0723) -> (-17.7588, -31.4498)
  spline S150 degree 2 poles (-17.7588, -31.4498) (-17.7588, -31.3484) (-17.6649, -31.2507) (-17.5748, -31.2507) knots 0 0 0 1 2 2 2
  line L58 (-17.5748, -31.2507) -> (-15.8133, -31.2507)
  spline S151 degree 2 poles (-15.8133, -31.2507) (-15.7907, -31.2507) (-15.7419, -31.277) (-15.7119, -31.3333) (-15.6969, -31.4197) (-15.6969, -31.4798) knots 0 0 0 1 2 3 4 4 4
  spline S152 degree 2 poles (-15.6969, -31.4798) (-15.6969, -31.5887) (-15.7569, -31.7127) (-15.8095, -31.7127) knots 0 0 0 1 2 2 2
  line L59 (-15.8095, -31.7127) -> (-17.2292, -31.7127)
  line L60 (-17.2292, -31.7127) -> (-17.2292, -32.8319)
  spline S153 degree 2 poles (-17.2292, -32.8319) (-17.1241, -32.8169) (-16.91, -32.8094) (-16.7673, -32.8094) knots 0 0 0 1 2 2 2
  spline S154 degree 2 poles (-16.7673, -32.8094) (-16.4368, -32.8094) (-15.9447, -32.9709) (-15.618, -33.2714) (-15.449, -33.6958) (-15.449, -33.9549) knots 0 0 0 1 2 3 4 4 4
  dimension "d19" = 9.25
  dimension "d20" = 9.5
  dimension "d21" = 9.75
  dimension "d22" = 10
  dimension "d23" = 10.25
  constraints: 10 other
  measures "d19" radius of A1
  measures "d20" radius of A2
  measures "d21" radius of A10
  measures "d22" radius of A7
  measures "d23" radius of A12
extrude "Выдавливание3" cut sketch "Эскиз3" against normal blind 1 contours S0 L20 S1 S2 L21 L22 L23 S3 S4 L24 S5 S6 L25 L26 S7 | S8 S9 S10 S11 S12 S13 S14 S15 | S24 S25 S26 S27 | S28 S29 S30 S31 S32 S33 S34 S35 L27 S36 L28 S37 S38 L29 L30 S39 S40 | S41 L31 S42 S43 L32 L33 L34 S44 S45 L35 S46 S47 L36 L37 S48 | S49 S50 S51 S52 S53 S54 S55 S56 S57 | S62 L38 S63 S64 L39 S65 S66 S67 S68 S69 S70 S71 L40 L41 S72 | S73 S74 S75 S76 | S81 L42 S82 S83 L43 L44 L45 S84 S85 L46 S86 S87 L47 L48 S88 | S89 S90 S91 S92 S93 S94 S95 S96 S97 | S102 S103 S104 S105 | S106 S107 S108 S109 S110 S111 S112 S113 L49 S114 L50 S115 S116 L51 L52 S117 S118 | S119 L53 S120 S121 L54 S122 S123 S124 S125 S126 S127 S128 L55 L56 S129 | S130 S131 S132 S133 | S138 S139 S140 S141 | S142 S143 S144 S145 S146 S147 S148 S149 L57 S150 L58 S151 S152 L59 L60 S153 S154
